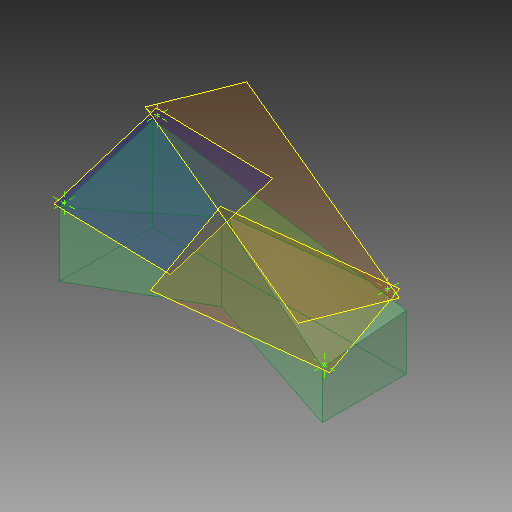
# Autodesk Inventor part: wall
Saved by Autodesk Inventor 2018.1 (Build 221171000, 171)
## iProperties
Created: 2017-10-14
Part Number: wall
Material: 一般
Document SubType Name: Modeling
Designer: formula
Density: 1 g/cm^3
Appearance: クリア - 緑 1
Author: formula
Autodesk Inventor part; units mm, degrees
ref_plane "YZ Plane" through (0, 0, 0) normal (1, 0, 0) x (0, 1, 0)
ref_plane "XZ Plane" through (0, 0, 0) normal (0, 1, 0) x (-1, 0, 0)
ref_plane "XY Plane" through (0, 0, 0) normal (0, 0, 1) x (1, 0, 0)
sketch "スケッチ5" plane through (0, 0, 0) normal (0, 1, 0) x (-1, 0, 0)
  line L0 (-559.0798, 16.0883) -> (-559.0798, -283.3342)
  line L1 (-559.0798, -283.3342) -> (344.6263, -283.3342)
  line L2 (344.6263, -283.3342) -> (344.6263, 47.8084)
  line L3 (-559.0798, 16.0883) -> (-22.4967, -162.5803)
  line L4 (-22.4967, -162.5803) -> (344.6263, 47.8084)
  point P0 (0, 0)
  constraints: 10 end point, 2 vertical, 1 perpendicular
extrude "押し出し5" add sketch "スケッチ5" along normal blind 360
sketch3d "3D スケッチ1"
ref_plane "作業平面1" through (557.1342, 171.5665, 5.3514) normal (0.1727, 0.9812, 0.0862) x (-0.2514, 0.1285, -0.9593)
ref_plane "作業平面4" through (-344.5976, 233.5337, 31.5954) normal (-0.0442, -0.9544, -0.2952) x (-0.0031, 0.2956, -0.9553)
ref_plane "作業平面5" through (-345.6786, 336.3426, -300.6801) normal (0.1489, 0.9888, -0.0028) x (0.9391, -0.1406, 0.3137)
sketch "スケッチ6" plane through (557.1342, 171.5665, 5.3514) normal (0.1727, 0.9812, 0.0862) x (-0.2514, 0.1285, -0.9593)
  line L0 (-514.7241, -766.6326) -> (967.6123, -766.6326)
  line L1 (967.6123, -766.6326) -> (967.6123, 1684.2947)
  line L2 (967.6123, 1684.2947) -> (-514.7241, 1684.2947)
  line L3 (-514.7241, 1684.2947) -> (-514.7241, -766.6326)
  point P0 (123.1359, 504.4343)
  constraints: 8 end point, 2 parallel, 1 horizontal, 1 perpendicular
sketch "スケッチ7" plane through (-345.6786, 336.3426, -300.6801) normal (0.1489, 0.9888, -0.0028) x (0.9391, -0.1406, 0.3137)
  line L0 (2221.5026, -667.2238) -> (-1676.0607, -667.2238)
  line L1 (-1676.0607, -667.2238) -> (-1676.0607, 746.6169)
  line L2 (-1676.0607, 746.6169) -> (2221.5026, 746.6169)
  line L3 (2221.5026, 746.6169) -> (2221.5026, -667.2238)
  point P0 (466.2154, -161.8023)
  constraints: 8 end point, 2 parallel, 1 horizontal, 1 perpendicular
sketch "スケッチ8" plane through (-344.5976, 233.5337, 31.5954) normal (-0.0442, -0.9544, -0.2952) x (-0.0031, 0.2956, -0.9553)
  line L0 (-1292.5456, 2575.2008) -> (1231.0674, 2575.2008)
  line L1 (1231.0674, 2575.2008) -> (1231.0674, -1866.358)
  line L2 (1231.0674, -1866.358) -> (-1292.5456, -1866.358)
  line L3 (-1292.5456, -1866.358) -> (-1292.5456, 2575.2008)
  point P0 (-39.9159, 354.4214)
  constraints: 8 end point, 2 parallel, 1 horizontal, 1 perpendicular
extrude "押し出し6" cut sketch "スケッチ7" along normal blind 360
extrude "押し出し7" cut sketch "スケッチ8" against normal blind 360
extrude "押し出し8" cut sketch "スケッチ6" along normal blind 360
